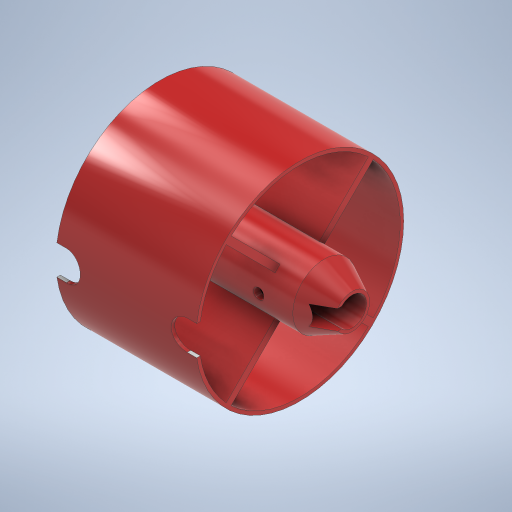
# Autodesk Inventor part: Tambor3
Saved by Autodesk Inventor 2023 (Build 270158000, 158)
## iProperties
Created: 2022-11-24
Part Number: Tambor3
Material: Genérico
Document SubType Name: Modeling
Designer: sergi
Density: 1 g/cm^3
Appearance: Valor por defecto
Author: sergi
Autodesk Inventor part; units mm, degrees
ref_plane "YZ Plane" through (0, 0, 0) normal (1, 0, 0) x (0, 1, 0)
ref_plane "XZ Plane" through (0, 0, 0) normal (0, 1, 0) x (-1, 0, 0)
ref_plane "XY Plane" through (0, 0, 0) normal (0, 0, 1) x (1, 0, 0)
ref_plane "Plano de trabajo3" through (185, 53, 51.5) normal (1, 0, 0) x (0, 0, -1)
ref_plane "Plano de trabajo4" through (125.2094, 54.5, 50) normal (1, 0, 0) x (0, 0, -1)
sketch "Boceto3" plane through (125.2094, 54.5, 50) normal (1, 0, 0) x (0, 0, -1)
  circle A0 centre (0, 0) radius 29.75
  circle A1 centre (0, 0) radius 5
  point P0 (50, -54.5)
  dimension "d5" = 59.5
  dimension "d9" = 10
  constraints: 2 centre point, 1 coincident
  measures "d5" diameter of A0
  measures "d9" diameter of A1
extrude "Extrusión1" add sketch "Boceto3" along normal blind 40 contours A0 | A1
shell "Vaciado1" thickness 1 removed faces 2 at (165.2094, 56.8732, 44.783) at (125.2094, 56.8732, 44.783)
sketch "Boceto4" plane through (165.2094, 54.5, 50) normal (1, 0, 0) x (0, 0, -1)
  circle A0 centre (0, 0) radius 9
  circle A1 centre (0, 0) radius 4.1
  point P0 (50, -54.5)
  dimension "d10" = 18
  dimension "d11" = 8.2
  constraints: 2 centre point, 1 coincident
  measures "d10" diameter of A0
  measures "d11" diameter of A1
extrude "Extrusión2" add sketch "Boceto4" against normal blind 40
sketch "Boceto5" plane through (165.2094, 54.5, 50) normal (1, 0, 0) x (0, 0, -1)
  line L0 (0, 0) -> (-4.1, 0)
  circle A0 centre (0, 0) radius 4.1 projected
  line L1 (-4.1, 0) -> (-7.1, 0)
  line L2 (-1.1, -2.8) -> (-7.1, -2.8)
  line L3 (-7.1, -2.8) -> (-7.1, 2.8)
  line L4 (-7.1, 2.8) -> (-1.1, 2.8)
  line L5 (-1.1, 2.8) -> (-1.1, -2.8)
  line L6 (-1.1, -2.8) -> (-7.1, 2.8) construction
  line L7 (-7.1, -2.8) -> (-1.1, 2.8) construction
  point P0 (50, -54.5)
  point P1 (-2.995, -2.8)
  point P2 (-2.995, 2.8)
  point P3 (-1.1, 0)
  dimension "d14" = 3
  dimension "d15" = 5.6
  constraints: 16 end point, 3 horizontal, 2 midpoint, 2 parallel, 1 perpendicular, 2 other
  measures "d14" distance of L0.end L1.end
  measures "d15" distance of L2.end L3.end
extrude "Extrusión3" cut sketch "Boceto5" against normal blind 5.5 contours L1 L3 L4 A0 | A0 L2 L3 L1
sketch "Boceto6" plane through (165.2094, 51.7, 57.1) normal (0, 0, -1) x (-1, 0, 0)
  line L0 (0, 0) -> (0, 5.6) projected
  line L1 (0, 0) -> (5.5, 0) projected
  line L2 (5.5, 0) -> (5.5, 5.6) projected
  line L3 (0, 5.6) -> (5.5, 5.6) projected
  line L4 (5.5, 0) -> (5.5, 5.6) projected
  line L5 (5.5, 5.6) -> (0, 0)
  circle A0 centre (2.75, 2.8) radius 1.5
  point P0 (165.2094, -51.7)
  dimension "d18" = 3
  constraints: 2 end point, 1 centre point, 1 midpoint
  measures "d18" diameter of A0
hole "Agujero1" at (162.4594, 54.5, 57.1) direction (0, 0, 1) diameter 3 depth 3.7 tip angle 118
ref_plane "Plano de trabajo5" through (145.2094, 54.5, 50) normal (1, 0, 0) x (0, 0, -1)
ref_plane "Plano de trabajo6" through (0, 0, 80) normal (0, 0, 1) x (1, 0, 0)
sketch "Boceto7" plane through (0, 0, 80) normal (0, 0, 1) x (1, 0, 0)
  line L0 (162.4594, 56) -> (162.4594, 53)
  arc A0 (162.4594, 58.75) -> (162.4594, 50.25) centre (162.4594, 54.5) ccw
  line L1 (162.4594, 58.75) -> (171.7607, 58.75)
  line L2 (171.7607, 58.75) -> (171.7607, 50.25)
  line L3 (171.7607, 50.25) -> (162.4594, 50.25)
  line L4 (125.2094, 50.4) -> (165.2094, 50.4) projected
  point P0 (0, 0)
  dimension "d27" = 8.5
  constraints: 8 end point, 2 point on circle, 1 centre point, 1 horizontal, 1 midpoint, 1 parallel, 1 perpendicular, 1 tangent, 1 vertical, 1 vertical alignment, 1 other
  measures "d27" diameter of A0
extrude "Extrusión4" cut sketch "Boceto7" against normal blind 5.5
mirror "Simetría2" about plane through (145.2094, 54.5, 50) normal (1, 0, 0) of "Extrusión4", "Agujero1", "Extrusión3"
sketch "Boceto10" plane through (165.2094, 54.5, 50) normal (1, 0, 0) x (0, 0, -1)
  line L0 (20.5061, -21.9203) -> (21.9203, -20.5061)
  line L1 (21.7316, -20.3174) -> (-20.3174, 21.7316)
  line L2 (-20.5061, 21.9203) -> (-21.9203, 20.5061)
  line L3 (-21.7316, 20.3174) -> (20.3174, -21.7316)
  line L4 (20.5061, -21.9203) -> (-20.3239, 21.7256) construction
  line L5 (21.7256, -20.3239) -> (-21.9203, 20.5061) construction
  line L6 (21.9203, 20.5061) -> (20.5061, 21.9203)
  line L7 (20.3174, 21.7316) -> (-21.7316, -20.3174)
  line L8 (-21.9203, -20.5061) -> (-20.5061, -21.9203)
  line L9 (-20.3174, -21.7316) -> (21.7316, 20.3174)
  line L10 (21.9203, 20.5061) -> (-21.7256, -20.3239) construction
  line L11 (20.3239, 21.7256) -> (-20.5061, -21.9203) construction
  line L12 (-2.995, -2.8) -> (-7.1, -2.8) projected
  line L13 (-7.1, -2.8) -> (-7.1, 2.8) projected
  line L14 (-7.1, 2.8) -> (-2.995, 2.8) projected
  arc A0 (-2.995, -2.8) -> (-2.995, 2.8) centre (0, 0) ccw projected
  circle A1 centre (0, 0) radius 9 projected
  circle A2 centre (0, 0) radius 9
  arc A3 (-28.4341, -4.25) -> (-28.4341, 4.25) centre (0, 0) ccw projected
  line L15 (-29.6711, 2.1651) -> (-28.6684, 2.1651) projected
  circle A4 centre (0, 0) radius 29.75
  point P0 (50, -54.5)
  point P1 (0, 0)
  point P2 (2.1045, 3.5187)
  point P3 (3.5187, 2.1045)
  point P4 (-2.1045, -3.5187)
  point P5 (-4.2142, -2.8)
  point P6 (-4.2142, 2.8)
  point P7 (-2.1045, 3.5187)
  point P8 (3.5187, -2.1045)
  point P9 (2.1045, -3.5187)
  point P10 (-28.6684, -2.1651)
  point P11 (-19.6099, 21.0241)
  point P12 (-21.0241, 19.6099)
  point P13 (-7.0317, 5.6174)
  point P14 (-5.6174, 7.0317)
  point P15 (21.0241, 19.6099)
  point P16 (19.6099, 21.0241)
  point P17 (5.6174, 7.0317)
  point P18 (7.0317, 5.6174)
  point P19 (19.6099, -21.0241)
  point P20 (21.0241, -19.6099)
  point P21 (7.0317, -5.6174)
  point P22 (5.6174, -7.0317)
  point P23 (-21.0241, -19.6099)
  point P24 (-19.6099, -21.0241)
  point P25 (-5.6174, -7.0317)
  point P26 (-7.0317, -5.6174)
  dimension "d30" = 2
  dimension "d31" = 60
  dimension "d32" = 2
  dimension "d33" = 60
  constraints: 24 end point, 4 parallel, 4 point on line, 2 coincident, 2 perpendicular, 1 centre point, 1 concentric, 15 other
  measures "d30" distance of L2.end L2.start
  measures "d31" distance of L2.start L0.end
  measures "d32" distance of L8.end L8.start
  measures "d33" distance of L8.start L6.end
extrude "Extrusión5" add sketch "Boceto10" against normal blind 40 contours A3 L3 A1 L1 | L9 A1 L7 A3 | A3 L7 A1 L9 | L1 A1 L3 A3
sketch "Boceto11" plane through (165.2094, 54.5, 50) normal (1, 0, 0) x (0, 0, -1)
  arc A0 (-5.6174, -7.0317) -> (5.6174, -7.0317) centre (0, 0) ccw projected
  circle A1 centre (0, 0) radius 9
  arc A2 (21.0241, -19.6099) -> (21.0241, 19.6099) centre (0, 0) ccw projected
  arc A3 (-29.4449, -4.25) -> (-29.4449, 4.25) centre (0, 0) ccw projected
  line L0 (-21.0241, 19.6099) -> (-7.0317, 5.6174) projected
  arc A4 (-7.0317, 5.6174) -> (-7.0317, -5.6174) centre (0, 0) ccw projected
  line L1 (-7.0317, -5.6174) -> (-21.0241, -19.6099) projected
  arc A5 (-19.6099, -21.0241) -> (19.6099, -21.0241) centre (0, 0) ccw projected
  arc A6 (21.0241, -19.6099) -> (21.0241, 19.6099) centre (0, 0) ccw projected
  line L2 (21.0241, -19.6099) -> (7.0317, -5.6174) projected
  arc A7 (7.0317, -5.6174) -> (7.0317, 5.6174) centre (0, 0) ccw projected
  line L3 (7.0317, 5.6174) -> (21.0241, 19.6099) projected
  arc A8 (-19.6099, -21.0241) -> (19.6099, -21.0241) centre (0, 0) ccw projected
  line L4 (-19.6099, -21.0241) -> (-5.6174, -7.0317) projected
  arc A9 (-5.6174, -7.0317) -> (5.6174, -7.0317) centre (0, 0) ccw projected
  line L5 (5.6174, -7.0317) -> (19.6099, -21.0241) projected
  line L6 (19.6099, 21.0241) -> (5.6174, 7.0317) projected
  arc A10 (5.6174, 7.0317) -> (-5.6174, 7.0317) centre (0, 0) ccw projected
  line L7 (-5.6174, 7.0317) -> (-19.6099, 21.0241) projected
  arc A11 (19.6099, 21.0241) -> (-19.6099, 21.0241) centre (0, 0) ccw projected
  line L8 (-2.995, -2.8) -> (-7.1, -2.8) projected
  line L9 (-7.1, -2.8) -> (-7.1, 2.8) projected
  line L10 (-7.1, 2.8) -> (-2.995, 2.8) projected
  arc A12 (-2.995, -2.8) -> (-2.995, 2.8) centre (0, 0) ccw projected
  line L11 (-21.0241, 19.6099) -> (-7.0317, 5.6174) projected
  arc A13 (-7.0317, 5.6174) -> (-7.0317, -5.6174) centre (0, 0) ccw projected
  line L12 (-7.0317, -5.6174) -> (-21.0241, -19.6099) projected
  arc A14 (-28.4341, -4.25) -> (-21.0241, -19.6099) centre (0, 0) ccw projected
  arc A15 (-29.4449, -4.25) -> (-29.4449, 4.25) centre (0, 0) ccw projected
  arc A16 (-21.0241, 19.6099) -> (-28.4341, 4.25) centre (0, 0) ccw projected
  line L13 (-28.4341, -4.25) -> (-29.4449, -4.25) projected
  line L14 (-29.4449, 4.25) -> (-28.4341, 4.25) projected
  line L15 (21.0241, -19.6099) -> (7.0317, -5.6174) projected
  arc A17 (7.0317, -5.6174) -> (7.0317, 5.6174) centre (0, 0) ccw projected
  line L16 (7.0317, 5.6174) -> (21.0241, 19.6099) projected
  line L17 (-19.6099, -21.0241) -> (-5.6174, -7.0317) projected
  arc A18 (-5.6174, -7.0317) -> (5.6174, -7.0317) centre (0, 0) ccw projected
  line L18 (5.6174, -7.0317) -> (19.6099, -21.0241) projected
  line L19 (19.6099, 21.0241) -> (5.6174, 7.0317) projected
  arc A19 (5.6174, 7.0317) -> (-5.6174, 7.0317) centre (0, 0) ccw projected
  line L20 (-5.6174, 7.0317) -> (-19.6099, 21.0241) projected
  arc A20 (19.6099, 21.0241) -> (-19.6099, 21.0241) centre (0, 0) ccw projected
  arc A21 (-28.4341, -4.25) -> (-21.0241, -19.6099) centre (0, 0) ccw projected
  line L21 (-28.4341, -4.25) -> (-29.4449, -4.25) projected
  line L22 (-29.4449, 4.25) -> (-28.4341, 4.25) projected
  arc A22 (-21.0241, 19.6099) -> (-28.4341, 4.25) centre (0, 0) ccw projected
  point P0 (50, -54.5)
  point P1 (5.6174, -7.0317)
  constraints: 3 other
ref_plane "Plano de trabajo8" through (180.2094, 7.3879, -6.6886) normal (-1, 0, 0) x (0, -0.3543782, 0.9351022)
extrude "Extrusión6" add sketch "Boceto11" along normal up to surface (15 mm away) contours A1 A0
chamfer "Chaflán1" distance 4 distance2 8 2 edges at (180.2094, 63.5, 50) (180.2094, 45.5, 50) measured on face at (180.2094, 46, 50) measured on face at (180.2094, 63, 50)
